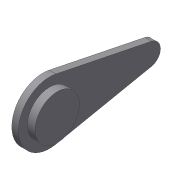
# Autodesk Inventor part: ANKLE_DRIVER_LOD
Saved by Autodesk Inventor 2019.4 (Build 234330000, 330)
## iProperties
Created: 2019-11-12
Part Number: ANKLE_DRIVER_LOD
Material: 一般
Document SubType Name: Modeling
Designer: y6tada
Density: 1 g/cm^3
Appearance: 既定
Author: y6tada
Autodesk Inventor part; units mm, degrees
ref_plane "YZ Plane" through (0, 0, 0) normal (1, 0, 0) x (0, 1, 0)
ref_plane "XZ Plane" through (0, 0, 0) normal (0, 1, 0) x (-1, 0, 0)
ref_plane "XY Plane" through (0, 0, 0) normal (0, 0, 1) x (1, 0, 0)
sketch "スケッチ1" plane through (0, 0, 0) normal (1, 0, 0) x (0, 1, 0)
  circle A0 centre (0, 0) radius 10
  line L0 (0, 0) -> (0, -45) construction
  arc A1 (0, -40) -> (-4.899, -46) centre (0, -45) ccw construction
  arc A2 (13.7171, -2.8) -> (-13.7171, -2.8) centre (0, 0) ccw
  line L1 (13.7171, -2.8) -> (4.899, -46)
  line L2 (-4.899, -46) -> (-13.7171, -2.8)
  arc A3 (0, -14) -> (13.7171, -2.8) centre (0, 0) ccw construction
  arc A4 (-13.7171, -2.8) -> (0, -14) centre (0, 0) ccw construction
  arc A5 (4.899, -46) -> (0, -40) centre (0, -45) ccw construction
  arc A6 (-4.899, -46) -> (4.899, -46) centre (0, -45) ccw
  dimension "d0" = 20
  dimension "d1" = 28
  dimension "d2" = 10
  dimension "d3" = 45
  constraints: 12 point on circle, 8 tangent, 7 centre point, 6 end point, 3 coincident, 2 point on line, 1 vertical
  measures "d0" diameter of A0
  measures "d1" diameter of A2
  measures "d2" diameter of A1
  measures "d3" distance of L0.start L0.end
extrude "押し出し1" add sketch "スケッチ1" along normal blind 3
sketch "スケッチ2" plane through (3, 0, 0) normal (1, 0, 0) x (0, 0, -1)
  circle A0 centre (0, 0) radius 7.5
  circle A1 centre (0, 0) radius 10 projected
  dimension "d7" = 15
  constraints: 1 centre point, 1 coincident
  measures "d7" diameter of A0
extrude "押し出し2" add sketch "スケッチ2" along normal blind 3.5 contours A0 | A1
sketch "スケッチ3" plane through (0, 0, 0) normal (-1, 0, 0) x (0, 0, 1)
  circle A0 centre (0, 0) radius 12 construction
  circle A1 centre (0, 0) radius 12.55
  circle A2 centre (0, 0) radius 11.45
  dimension "d10" = 24
  dimension "d11" = 0.55
  dimension "d12" = 0.55
  constraints: 3 centre point, 1 coincident
  measures "d10" diameter of A0
  measures "d11" radial gap between concentric circles of A2 A0
  measures "d12" radial gap between concentric circles of A0 A1
extrude "押し出し3" cut sketch "スケッチ3" against normal blind 0.25
